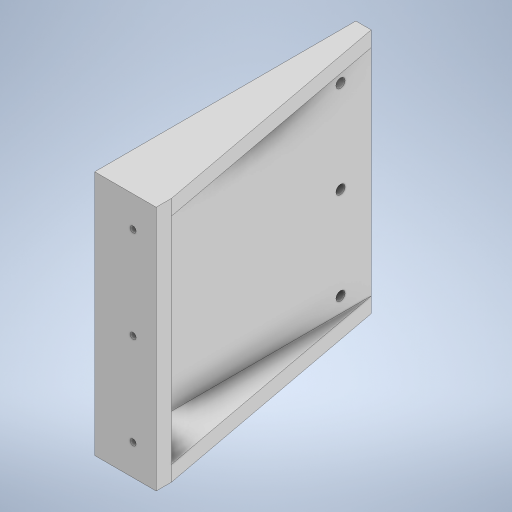
# Autodesk Inventor part: bracket_v02
Saved by Autodesk Inventor 2023 (Build 270158000, 158)
## iProperties
Created: 2021-04-13
Part Number: bracket_v02
Material: Generic
Document SubType Name: Modeling
Designer: KAMPFF-LAB-BEHAVIOR
Density: 1 g/cm^3
Appearance: Default
Author: KAMPFF-LAB-BEHAVIOR
Autodesk Inventor part; units mm, degrees
ref_plane "YZ Plane" through (0, 0, 0) normal (1, 0, 0) x (0, 1, 0)
ref_plane "XZ Plane" through (0, 0, 0) normal (0, 1, 0) x (-1, 0, 0)
ref_plane "XY Plane" through (0, 0, 0) normal (0, 0, 1) x (1, 0, 0)
sketch "Sketch21" plane through (0, 0, 0) normal (0, 0, 1) x (1, 0, 0)
  line L0 (0, 0) -> (30, 0)
  line L1 (30, 0) -> (30, -160)
  line L2 (30, -160) -> (0, -160)
  line L3 (0, -160) -> (0, 0)
  dimension "d53" = 30
  dimension "d1" = 160
  constraints: 8 end point, 2 parallel, 1 horizontal, 1 perpendicular
  measures "d53" distance of L1.end L2.end
  measures "d1" distance of L0.end L1.end
extrude "Extrusion15" add sketch "Sketch21" along normal blind 10
sketch "Sketch22" plane through (0, -160, 0) normal (-1, 0, 0) x (0, 0, 1)
  line L0 (0, 160) -> (10, 160) projected
  line L1 (10, 160) -> (-160, 160)
  line L2 (-160, 160) -> (-160, 0)
  line L3 (-160, 0) -> (10, 0)
  line L4 (10, 0) -> (10, 160)
  dimension "d57" = 170
  dimension "d58" = 160
  constraints: 8 end point, 2 parallel, 1 horizontal, 1 perpendicular
  measures "d57" distance of L3.end L2.end
  measures "d58" distance of L2.end L1.end
extrude "Extrusion16" add sketch "Sketch22" along normal blind 10
sketch "Sketch23" plane through (30, 0, 10) normal (0, 1, 0) x (1, 0, 0)
  line L0 (-30, 170) -> (-40, 170) projected
  line L1 (0, 10) -> (0, 0) projected
  line L2 (-30, 170) -> (0, 10)
  line L3 (-30, 10) -> (0, 10) projected
  line L4 (0, 10) -> (-30, 10)
  line L5 (-30, 10) -> (-30, 170)
  line L6 (-40, 170) -> (-40, 0) projected
  constraints: 6 end point, 1 collinear, 1 parallel
extrude "Extrusion17" add sketch "Sketch23" against normal blind 10
sketch "Sketch24" plane through (30, -160, 0) normal (0, -1, 0) x (1, 0, 0)
  line L0 (-30, -160) -> (-40, -160) projected
  line L1 (-30, 0) -> (0, 0) projected
  line L2 (-30, -160) -> (-30, 0)
  line L3 (0, 0) -> (0, 10) projected
  line L4 (-30, 0) -> (0, 0)
  line L5 (-30, -160) -> (0, 0) projected
  line L6 (0, 0) -> (-30, -160)
  constraints: 6 end point, 1 collinear, 1 perpendicular, 1 vertical
extrude "Extrusion18" add sketch "Sketch24" against normal blind 10
sketch "Sketch25" plane through (0, 0, 10) normal (0, 0, 1) x (1, 0, 0)
  circle A0 centre (15, -20) radius 2
  circle A1 centre (15, -80) radius 2
  circle A2 centre (15, -140) radius 2
  line L0 (30, -160) -> (-10, -160) projected
  line L1 (30, 0) -> (-10, 0) projected
  point P0 (0, 0)
  dimension "d65" = 4
  dimension "d66" = 4
  dimension "d67" = 4
  dimension "d70" = 20
  dimension "d71" = 20
  dimension "d72" = 80
  constraints: 3 centre point
  measures "d65" diameter of A0
  measures "d66" diameter of A1
  measures "d67" diameter of A2
  measures "d70" distance from line of A2.centre L0
  measures "d71" distance from line of A0.centre L1
  measures "d72" distance from line of A1.centre L0
extrude "Extrusion19" cut sketch "Sketch25" against normal blind 20
sketch "Sketch27" plane through (-10, -160, 0) normal (-1, 0, 0) x (0, 0, 1)
  circle A0 centre (-10, 20) radius 3
  line L0 (-160, 0) -> (10, 0) projected
  circle A1 centre (-10, 80) radius 3
  circle A2 centre (-10, 140) radius 3
  line L1 (10, 160) -> (-160, 160) projected
  line L2 (10, 0) -> (10, 160) projected
  circle A3 centre (-140, 80) radius 3
  line L3 (-160, 160) -> (-160, 0) projected
  circle A4 centre (-140, 20) radius 3
  circle A5 centre (-140, 140) radius 3
  point P0 (0, 160)
  dimension "d73" = 20
  dimension "d74" = 6
  dimension "d75" = 6
  dimension "d76" = 80
  dimension "d77" = 6
  dimension "d78" = 20
  dimension "d79" = 20
  dimension "d80" = 20
  dimension "d81" = 20
  dimension "d84" = 6
  dimension "d85" = 20
  dimension "d86" = 80
  dimension "d87" = 6
  dimension "d88" = 20
  dimension "d89" = 20
  dimension "d90" = 6
  dimension "d91" = 20
  dimension "d92" = 20
  constraints: 6 centre point
  measures "d73" distance from line of A0.centre L0
  measures "d74" diameter of A0
  measures "d75" diameter of A1
  measures "d76" distance from line of A1.centre L0
  measures "d77" diameter of A2
  measures "d78" distance from line of A2.centre L1
  measures "d79" distance from line of A1.centre L2
  measures "d80" distance from line of L2 A2.centre
  measures "d81" distance from line of L2 A0.centre
  measures "d84" diameter of A3
  measures "d85" distance from line of A3.centre L3
  measures "d86" distance from line of A3.centre L0
  measures "d87" diameter of A4
  measures "d88" distance from line of A4.centre L3
  measures "d89" distance from line of L0 A4.centre
  measures "d90" diameter of A5
  measures "d91" distance from line of A5.centre L3
  measures "d92" distance from line of A5.centre L1
extrude "Extrusion20" cut sketch "Sketch27" against normal blind 20 contours A0 | A1 | A2 | A3 | A4 | A5
sketch "Sketch29" plane through (-10, -160, 0) normal (-1, 0, 0) x (0, 0, 1)
  circle A0 centre (-140, 80) radius 3 projected
  circle A1 centre (-140, 80) radius 5
  circle A2 centre (-140, 20) radius 3 projected
  circle A3 centre (-140, 20) radius 5
  circle A4 centre (-140, 140) radius 3 projected
  circle A5 centre (-140, 140) radius 5
  circle A6 centre (-10, 20) radius 3 projected
  circle A7 centre (-10, 20) radius 5
  circle A8 centre (-10, 80) radius 3 projected
  circle A9 centre (-10, 80) radius 5
  circle A10 centre (-10, 140) radius 3 projected
  circle A11 centre (-10, 140) radius 5
  point P0 (0, 160)
  dimension "d93" = 10
  dimension "d94" = 10
  dimension "d95" = 10
  dimension "d96" = 10
  dimension "d97" = 10
  dimension "d98" = 10
  constraints: 6 centre point, 6 coincident
  measures "d93" diameter of A1
  measures "d94" diameter of A3
  measures "d95" diameter of A5
  measures "d96" diameter of A7
  measures "d97" diameter of A9
  measures "d98" diameter of A11
extrude "Extrusion21" cut sketch "Sketch29" against normal blind 4 contours A0 | A1 | A2 | A3 | A4 | A5 | A6 | A7 | A8 | A9 | A10 | A11
equation "\"d58\" = d1"
equation "\"d65\" = d67"
equation "\"d66\" = d67"
equation "\"d71\" = d70"
equation "\"d73\" = d70"
equation "\"d74\" = d75"
equation "\"d76\" = d72"
equation "\"d77\" = d75"
equation "\"d78\" = d70"
equation "\"d80\" = d79"
equation "\"d81\" = d79"
equation "\"d84\" = d75"
equation "\"d85\" = d79"
equation "\"d86\" = d72"
equation "\"d87\" = d75"
equation "\"d88\" = d79"
equation "\"d89\" = d70"
equation "\"d90\" = d75"
equation "\"d91\" = d79"
equation "\"d92\" = d70"
equation "\"d94\" = d93"
equation "\"d95\" = d93"
equation "\"d96\" = d93"
equation "\"d97\" = d93"
equation "\"d98\" = d93"
body "Solid5"
